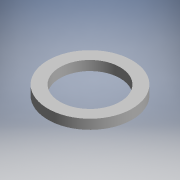
# Autodesk Inventor part: 247465 FEN-80-SD---(SD)
Saved by Autodesk Inventor 2017.3 (Build 213256000, 256)
## iProperties
Part Number: 247465 FEN-80-SD---(SD)
Material: Generic
Catalog Web Link: www.cadenas.de
Description: FEN-X-(SD)-Abstreifer
Vendor: FESTO
Document SubType Name: Modeling
Designer: partserver
Manufacturer: FESTO
Mass: 1.57795 g
Surface Area: 18.0904 cm^2
Volume: 1.57795 cm^3
Density: 1 g/cm^3
Appearance: PSOLRGB-224-224-224
Category: PARTsolutions
Company: FESTO
Title: 247465 FEN-80-SD---(SD)
Author: Cadenas PARTsolutions
Comments: Abstreifer
PSOL_IDENT_0: {$CADENAS_DATA\23d-libs\festo\parts\e\eagf\parts\eagf_abstreif.prj},190 {VTYP=3D},{NB=247465 FEN-80-
PSOL_IDENT_1: SD---(SD)},{LINA=247465 FEN-80-SD---(SD)},{NN=FEN-X-(SD)},{DATE=20.07.2020 13:53:58},{GEOMDATE=02.09
PSOL_IDENT_2: .2015 14:27:16},{VERSION=},{LINEID=20},{WBVAR=},{WBNUMERIC=}  {NB=247465 FEN-80-SD---(SD)},{LINA=247
PSOL_IDENT_3: 465 FEN-80-SD---(SD)},{KT=DUMMY},{TNR=247465},{TYP=FEN-80-SD},{D1=35.000},{D2=25.000},{B=4.000}
NB: 247465 FEN-80-SD---(SD)
NN: FEN-X-(SD)
NT: Abstreifer
NBSYN: $TNR. $TYP.---(SD)
LINA: 247465 FEN-80-SD---(SD)
CATALOG: Festo
TNR: 247465
TYP: FEN-80-SD
D1: 35
D2: 25
B: 4
SUPPLIER: FESTO
ARTICLENO: 247465 FEN-80-SD---(SD)
BOMINFO: 247465 FEN-80-SD---(SD)
CREATOR: CADENAS GmbH
Autodesk Inventor part; units mm, degrees
sketch "Sketch_1" plane through (0, 0, 0) normal (1, 0, 0) x (0, 1, 0)
  line L0 (0, -4) -> (0, 0)
  line L1 (12.5, 0) -> (12.5, -4)
  line L2 (12.5, -4) -> (17.5, -4)
  line L3 (17.5, -4) -> (17.5, 0)
  line L4 (17.5, 0) -> (16.4679, 0)
  line L5 (16.4679, 0) -> (16.2, -1)
  line L6 (16.2, -1) -> (13.5, -1)
  line L7 (13.5, -1) -> (12.5, 0)
  constraints: 16 end point
revolve "Revolution1" add sketch "Sketch_1" angle 360 about axis through (0, 0, -4) along (0, 0, -1)
ref_plane "ANBAU_XY" through (0, 0, -4) normal (0, 0, 1) x (1, 0, 0)
ref_plane "ANBAU_YZ" through (0, 0, -4) normal (1, 0, 0) x (0, 1, 0)
ref_plane "ANBAU_ZX" through (0, 0, -4) normal (0, 1, 0) x (0, 0, 1)
body "Solid1"
